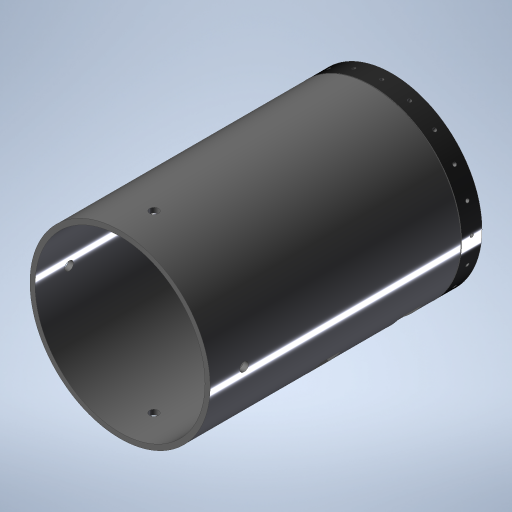
# Autodesk Inventor part: Avionics and Recovery
Saved by Autodesk Inventor 2023 (Build 270158000, 158)
## iProperties
Created: 2022-01-31
Part Number: Avionics and Recovery
Material: GFRC
Document SubType Name: Modeling
Designer: boleh
Density: 1.7 g/cm^3
Appearance: White
Mass: 1387.33 g
Surface Area: 6610.55 cm^2
Volume: 816.078 cm^3
Author: boleh
Autodesk Inventor part; units mm, degrees
sketch "Sketch1" plane through (0, 0, 0) normal (0, 0, 1) x (1, 0, 0)
  circle A0 centre (0, 0) radius 132.5
  circle A1 centre (0, 0) radius 125
  dimension "d0" = 265
  dimension "d1" = 250
  constraints: 2 centre point, 2 coincident
  measures "d0" diameter of A0
  measures "d1" diameter of A1
extrude "Extrusion1" add sketch "Sketch1" against normal blind 400
ref_plane "Work Plane1" through (0, 0, -370) normal (0, 0, -1) x (-1, 0, 0)
sketch "Sketch3" plane through (0, 0, -370) normal (0, 0, -1) x (-1, 0, 0)
  circle A0 centre (0, 0) radius 125 projected
  circle A1 centre (0, 0) radius 132.5 projected
  circle A2 centre (0, 0) radius 131.5
  dimension "d27" = 1
  constraints: 1 centre point, 1 coincident
  measures "d27" radial gap between concentric circles of A1 A2
extrude "Extrusion3" cut sketch "Sketch3" against normal blind 1 contours A1
ref_plane "Work Plane2" through (132.5, 0, 0) normal (1, 0, 0) x (0, 1, 0)
sketch "Sketch4" plane through (132.5, 0, 0) normal (1, 0, 0) x (0, 1, 0)
  circle A0 centre (0, -385) radius 2.5
  line L0 (-132.5, -400) -> (132.5, -400) projected
  point P0 (0, 0)
  dimension "d30" = 15
  dimension "d31" = 5
  constraints: 1 centre point
  measures "d30" distance from line of L0 A0.centre
  measures "d31" diameter of A0
extrude "Extrusion4" cut sketch "Sketch4" against normal blind 30
pattern_circular "Circular Pattern2" count 20 over 360 about axis through (0, 0, 0) along (0, 0, -1) of "Extrusion4"
ref_plane "Work Plane4" through (101.5009, -85.1694, 0) normal (-0.766, 0.6428, 0) x (0, 0, 1)
ref_plane "Work Plane3" through (0, 0, 0) normal (-0.766, 0.6428, 0) x (0, 0, 1)
sketch "Sketch8" plane through (101.5009, -85.1694, 0) normal (-0.766, 0.6428, 0) x (0, 0, 1)
  line L0 (-303.5, -11.25) -> (-336.5, -11.25)
  line L1 (-336.5, -11.25) -> (-336.5, 11.25)
  line L2 (-336.5, 11.25) -> (-303.5, 11.25)
  line L3 (-303.5, 11.25) -> (-303.5, -11.25)
  line L4 (-303.5, -11.25) -> (-336.5, 11.25) construction
  line L5 (-336.5, -11.25) -> (-303.5, 11.25) construction
  line L6 (0, 132.5) -> (0, -132.5) projected
  line L7 (-310, -27.25) -> (-330, -27.25)
  line L8 (-330, -27.25) -> (-330, -13.25)
  line L9 (-330, -13.25) -> (-310, -13.25)
  line L10 (-310, -13.25) -> (-310, -27.25)
  line L11 (-310, -27.25) -> (-330, -13.25) construction
  line L12 (-330, -27.25) -> (-310, -13.25) construction
  line L13 (-320, 0) -> (-320, -6.921)
  line L14 (-303.5, -13.25) -> (-310, -13.25)
  line L15 (-310, -13.25) -> (-310, -27.25)
  line L16 (-310, -27.25) -> (-303.5, -27.25)
  line L17 (-303.5, -27.25) -> (-303.5, -13.25)
  line L18 (-303.5, -13.25) -> (-310, -27.25) construction
  line L19 (-310, -13.25) -> (-303.5, -27.25) construction
  line L20 (-336.5, -13.25) -> (-330, -13.25)
  line L21 (-330, -13.25) -> (-330, -27.25)
  line L22 (-330, -27.25) -> (-336.5, -27.25)
  line L23 (-336.5, -27.25) -> (-336.5, -13.25)
  line L24 (-336.5, -13.25) -> (-330, -27.25) construction
  line L25 (-330, -13.25) -> (-336.5, -27.25) construction
  line L26 (-185, 15) -> (-215, 15)
  line L27 (-215, 15) -> (-215, -15)
  line L28 (-215, -15) -> (-185, -15)
  line L29 (-185, -15) -> (-185, 15)
  line L30 (-185, 15) -> (-215, -15) construction
  line L31 (-215, 15) -> (-185, -15) construction
  point P0 (0, 0)
  point P1 (0, 0)
  point P2 (-320, -20.25)
  point P3 (-306.75, -20.25)
  point P4 (-333.25, -20.25)
  point P5 (-200, 0)
  dimension "d52" = 33
  dimension "d53" = 320
  dimension "d54" = 22.5
  dimension "d57" = 20
  dimension "d58" = 14
  dimension "d59" = 2
  dimension "d68" = 6.5
  dimension "d69" = 14
  dimension "d70" = 30
  dimension "d71" = 30
  dimension "d72" = 200
  constraints: 62 end point, 11 midpoint, 10 parallel, 5 horizontal, 5 perpendicular, 4 horizontal alignment, 3 point on line, 2 equal length, 1 vertical, 1 vertical alignment
  measures "d52" distance of L0.start L0.end
  measures "d53" distance from line of L6 L13.start
  measures "d54" distance of L2.end L0.start
  measures "d57" distance of L7.start L7.end
  measures "d58" distance of L9.end L7.start
  measures "d59" distance between parallel lines of L0 L9
  measures "d68" distance of L14.start L14.end
  measures "d69" distance of L16.end L14.start
  measures "d70" distance of L26.start L26.end
  measures "d71" distance of L26.end L27.end
  measures "d72" distance from line of L6 point (-200, 0)
extrude "Extrusion7" cut sketch "Sketch8" along normal blind 10
sketch "Sketch9" plane through (101.5009, -85.1694, 0) normal (-0.766, 0.6428, 0) x (0, 0, 1)
  line L0 (-303.5, 11.25) -> (-336.5, 11.25)
  line L1 (-336.5, 11.25) -> (-336.5, -28.75)
  line L2 (-336.5, -28.75) -> (-303.5, -28.75)
  line L3 (-303.5, -28.75) -> (-303.5, 11.25)
  line L4 (-303.5, 11.25) -> (-336.5, -28.75) construction
  line L5 (-336.5, 11.25) -> (-303.5, -28.75) construction
  line L6 (-303.5, 11.25) -> (-336.5, 11.25) projected
  point P0 (0, 0)
  point P1 (-320, -8.75)
  point P2 (-320, 11.25)
  dimension "d76" = 40
  dimension "d77" = 33
  constraints: 12 end point, 4 midpoint, 2 parallel, 1 horizontal, 1 perpendicular
  measures "d76" distance of L0.end L1.end
  measures "d77" distance between parallel lines of L1 L3
extrude "Extrusion8" cut sketch "Sketch9" along normal blind 10
sketch "Sketch10" plane through (0, 0, 0) normal (0, 1, 0) x (-1, 0, 0)
  circle A0 centre (0, -50) radius 6.5
  line L0 (-132.5, 0) -> (132.5, 0) projected
  point P0 (0, 0)
  dimension "d78" = 13
  dimension "d79" = 50
  constraints: 1 centre point
  measures "d78" diameter of A0
  measures "d79" distance from line of L0 A0.centre
extrude "Extrusion9" cut sketch "Sketch10" against normal through all
pattern_circular "Circular Pattern3" count 4 over 360 about axis through (0, 0, 0) along (0, 0, -1) of "Extrusion9"
body "Solid1"
